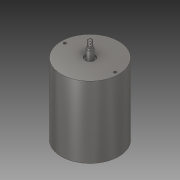
# Autodesk Inventor part: boma_2kw_motor
Saved by Autodesk Inventor 2019 (Build 230136000, 136)
## iProperties
Created: 2018-09-22
Part Number: boma_2kw_motor
Material: Steel, Mild
Document SubType Name: Modeling
Designer: Callum Snowden
Mass: 9645.45 g
Surface Area: 661.659 cm^2
Volume: 1228.72 cm^3
Density: 7.85 g/cm^3
Appearance: Semi-Polished
Author: Callum Snowden
Autodesk Inventor part; units mm, degrees
ref_plane "YZ Plane" through (0, 0, 0) normal (1, 0, 0) x (0, 1, 0)
ref_plane "XZ Plane" through (0, 0, 0) normal (0, 1, 0) x (-1, 0, 0)
ref_plane "XY Plane" through (0, 0, 0) normal (0, 0, 1) x (1, 0, 0)
sketch "Sketch1" plane through (0, 0, 0) normal (0, 1, 0) x (-1, 0, 0)
  circle A0 centre (0, 0) radius 54
  dimension "d0" = 108
  constraints: 1 centre point, 1 coincident
  measures "d0" diameter of A0
extrude "Extrusion1" add sketch "Sketch1" along normal blind 134
sketch "Sketch2" plane through (0, 134, 0) normal (0, 1, 0) x (1, 0, 0)
  circle A0 centre (0, 0) radius 9
  dimension "d3" = 18
  constraints: 1 centre point, 1 coincident
  measures "d3" diameter of A0
extrude "Extrusion2" cut sketch "Sketch2" against normal blind 2.5
sketch "Sketch3" plane through (0, 131.5, 0) normal (0, 1, 0) x (1, 0, 0)
  circle A0 centre (0, 0) radius 6
  dimension "d6" = 12
  constraints: 1 centre point, 1 coincident
  measures "d6" diameter of A0
extrude "Extrusion3" add sketch "Sketch3" along normal blind 17
sketch "Sketch4" plane through (0, 148.5, 0) normal (0, 1, 0) x (1, 0, 0)
  line L0 (-4.25, -2.6339) -> (-4.25, 2.6339)
  line L1 (4.25, -2.6339) -> (4.25, 2.6339)
  arc A0 (-4.25, -2.6339) -> (4.25, -2.6339) centre (0, 0) ccw
  arc A1 (4.25, 2.6339) -> (-4.25, 2.6339) centre (0, 0) ccw
  dimension "d10" = 8.5
  constraints: 4 end point, 4 point on circle, 2 centre point, 1 coincident, 1 parallel, 1 vertical
  measures "d10" distance between parallel lines of L1 L0
extrude "Extrusion4" add sketch "Sketch4" along normal blind 3.5
sketch "Sketch5" plane through (0, 134, 0) normal (0, 1, 0) x (1, 0, 0)
  line L0 (75.6, 0) -> (-75.6, 0) construction
  line L1 (0, 75.6) -> (0, -75.6) construction
  point P0 (0, 0)
  point P1 (-47.25, 0)
  point P2 (47.25, 0)
  dimension "d16" = 94.5
  constraints: 2 point on line, 1 symmetric about line
  measures "d16" distance of point (-47.25, 0) point (47.25, 0)
hole "Hole1" at (-47.25, 134, 0) at (47.25, 134, 0) direction (0, -1, 0) diameter 4.917 depth 10 tip angle 118 thread size "M6x1" class "6H" standard "ISO Metric profile"
sketch "Sketch6" plane through (0, 0, 0) normal (0, -1, 0) x (1, 0, 0)
  circle A0 centre (47.25, 0) radius 2.4585
  circle A1 centre (-47.25, 0) radius 2.4585
  line L0 (0, 75.6) -> (0, -75.6) construction
  point P0 (0, 0)
  dimension "d24" = 94.5
  constraints: 2 centre point, 1 symmetric about line
  measures "d24" distance of A1.centre A0.centre
hole "Hole2" at (47.25, 0, 0) at (-47.25, 0, 0) direction (0, 1, 0) diameter 4.917 depth 10 tip angle 118 thread size "M6x1" class "6H" standard "ISO Metric profile"
sketch "Sketch7" plane through (0, 152, 0) normal (0, 1, 0) x (1, 0, 0)
  circle A0 centre (0, 0) radius 4
  dimension "d32" = 8
  constraints: 1 centre point, 1 coincident
  measures "d32" diameter of A0
extrude "Extrusion5" add sketch "Sketch7" along normal blind 10.5
thread "Thread1" size "M8x1.25" class "6g" standard "ISO Metric profile" full length
sketch "Sketch9" plane through (0, 162.5, 0) normal (1, 0, 0) x (0, 0, 1)
  line L0 (4, 0) -> (4, 10.5)
  line L1 (4, 10.5) -> (3.0732, 10.5)
  line L2 (3.0732, 10.5) -> (3.0732, 0)
  line L3 (3.0732, 0) -> (4, 0)
  line L4 (0, -34.1357) -> (0, 195.2726) projected
  constraints: 8 end point
revolve "Revolution1" cut sketch "Sketch9" angle 360 about axis through (0, 162.5, 0) along (0, -1, 0)
sketch "Sketch10" plane through (0, 162.5, 0) normal (1, 0, 0) x (0, 0, 1)
  line L0 (4, 0) -> (4, 10.5)
  line L1 (4, 10.5) -> (3.0732, 10.5)
  line L2 (3.0732, 10.5) -> (3.0732, 0)
  line L3 (3.0732, 0) -> (4, 0)
  line L4 (0, -34.1357) -> (0, 195.2726) projected
  constraints: 8 end point
revolve "Revolution2" add sketch "Sketch10" angle 360 about axis through (0, 162.5, 0) along (0, -1, 0) separate body
sketch "Sketch8" plane through (0, 162.5, 0) normal (-1, 0, 0) x (0, -1, 0)
  line L0 (-0.7293, -3.1366) -> (-0.6251, -3.1366) construction
  line L1 (0.1041, -3.937) -> (-0.0001, -4.1371) construction
  line L2 (-1.2501, -4.1371) -> (-1.3543, -3.937) construction
  line L3 (-0.5209, -3.1366) -> (-0.6251, -2.9364) construction
  line L4 (-0.6251, -2.9364) -> (-0.7293, -3.1366) construction
  line L5 (-1.2501, -4.1371) -> (-1.1459, -3.937) construction
  line L6 (-0.5209, -3.1366) -> (-0.1043, -3.937)
  line L7 (-1.3543, -3.937) -> (-1.1459, -3.937) construction
  arc A0 (-1.3543, -3.937) -> (-1.2501, -4.0002) centre (-1.2501, -3.8827) ccw construction
  line L8 (0.1041, -3.937) -> (-0.1043, -3.937) construction
  line L9 (-1.2501, -4.1371) -> (-1.2501, -3.937) construction
  line L10 (-0.0001, -4.1371) -> (-0.0001, -3.937) construction
  line L11 (-0.6251, -2.9364) -> (-0.6251, -3.0733) construction
  line L12 (-1.2501, -4.0002) -> (-0.0001, -4.0002)
  arc A1 (-1.2501, -4.0002) -> (-1.1459, -3.937) centre (-1.2501, -3.8827) ccw
  line L13 (-0.1043, -3.937) -> (-0.0001, -4.1371) construction
  line L14 (-1.1459, -3.937) -> (-0.7293, -3.1366)
  line L15 (-0.0001, -0.0002) -> (-0.0001, 0.0177)
  line L16 (-0.0001, 0.0177) -> (-0.0001, -0.0002)
  line L17 (-0.0001, -0.0002) -> (0.0334, -0.0002)
  arc A2 (-0.1043, -3.937) -> (-0.0001, -4.0002) centre (-0.0001, -3.8827) ccw
  arc A3 (-0.0001, -4.0002) -> (0.1041, -3.937) centre (-0.0001, -3.8827) ccw construction
  arc A4 (-0.6251, -3.0733) -> (-0.7293, -3.1366) centre (-0.6251, -3.1908) ccw
  arc A5 (-0.5209, -3.1366) -> (-0.6251, -3.0733) centre (-0.6251, -3.1908) ccw
  line L18 (-0.6251, -3.0733) -> (-0.6251, -3.1366) construction
  line L19 (-0.6251, -3.1366) -> (-0.5209, -3.1366) construction
  dimension "d37" = 55
  dimension "d38" = 0.2001
  dimension "d39" = 0.2001
  dimension "Sketch8_ThreadOffset" = 0
  dimension "Sketch8_MajorRadius" = 4
  dimension "d42" = 1.25
  dimension "Sketch8_MinorRadius" = 3.0732
  constraints: 40 end point, 12 point on circle, 10 parallel, 8 tangent, 6 centre point, 6 collinear, 2 midpoint, 2 point on line, 1 horizontal, 1 perpendicular, 3 other
  measures "d37" angle of L6 L14
  measures "d38" distance of L3.end L0.end
  measures "d39" distance of L1.end L10.end
  measures "Sketch8_ThreadOffset" distance between parallel lines of L15 L10
  measures "Sketch8_MajorRadius" distance from line of L12 L15.start
  measures "d42" distance from line of L1.end L9
  measures "Sketch8_MinorRadius" distance edge to line of A5 L17
coil "Coil1" sketch "Sketch8" operation cut axis through (0, 162.5, 0) along (0, -1, 0) pitch 1.2513 turns 10.38961 hand left bodies 2
equation "\"d37\" = d44"
equation "\"d38\" = 0.160083 * Sketch8_Pitch"
equation "\"d39\" = 0.160083 * Sketch8_Pitch"
equation "\"d42\" = Sketch8_Pitch"
equation "\"d44\" = 55deg"
equation "\"Sketch8_Pitch\" = 1.25"
body "Solid1"
body "Solid2"
